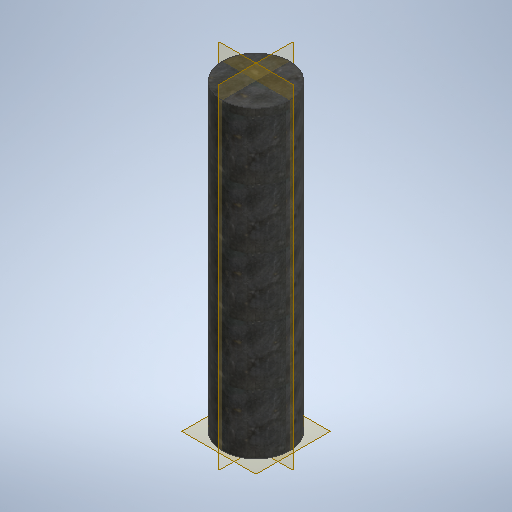
# Autodesk Inventor part: Z
Saved by Autodesk Inventor 2025.2 (Build 292293000, 293)
## iProperties
Created: 2025-03-23
Part Number: Z
Material: Steel
Document SubType Name: Modeling
Designer: MSIGAMING
Mass: 221954 g
Surface Area: 6283.19 cm^2
Volume: 28274.3 cm^3
Density: 7.85 g/cm^3
Appearance: Plate
Author: MSIGAMING
Autodesk Inventor part; units mm, degrees
sketch "Sketch1" plane through (0, 0, 0) normal (0, 1, 0) x (-1, 0, 0)
  circle A0 centre (0, 0) radius 100
  dimension "d0" = 200
  constraints: 1 centre point, 1 coincident
  measures "d0" diameter of A0
extrude "Extrusion1" add sketch "Sketch1" along normal blind 900
body "Solid1"
